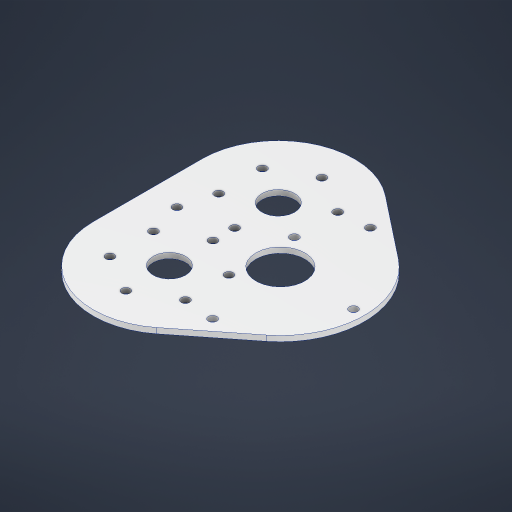
# Autodesk Inventor part: Gearboxes_3_thingy that holds motors and more
Saved by Autodesk Inventor 2024.4 (Build 284460000, 460)
## iProperties
Created: 2026-06-11
Part Number: Gearboxes_3_thingy that holds motors and more
Material: Aluminum 6061
Document SubType Name: Modeling
Designer: stanr
Density: 2.7 g/cm^3
Appearance: Aluminum - Flat
Author: stanr
Autodesk Inventor part; units mm, degrees
ref_plane "YZ Plane" through (0, 0, 0) normal (1, 0, 0) x (0, 1, 0)
ref_plane "XZ Plane" through (0, 0, 0) normal (0, 1, 0) x (-1, 0, 0)
ref_plane "XY Plane" through (0, 0, 0) normal (0, 0, 1) x (1, 0, 0)
sketch "Sketch1" plane through (0, 0, 0) normal (0, 1, 0) x (-1, 0, 0)
  circle A0 centre (0, 0) radius 31.75 construction
  circle A1 centre (0, -63.5) radius 31.75 construction
  circle A2 centre (0, 0) radius 9.525
  circle A3 centre (0, -63.5) radius 9.525
  circle A4 centre (0, 0) radius 25.4 construction
  circle A5 centre (0, -63.5) radius 25.4 construction
  circle A6 centre (0, 25.4) radius 2.4892
  circle A7 centre (-21.997, 12.7) radius 2.4892
  circle A8 centre (-21.997, -12.7) radius 2.4892
  circle A9 centre (0, -25.4) radius 2.4892
  circle A10 centre (21.997, -12.7) radius 2.4892
  circle A11 centre (21.997, 12.7) radius 2.4892
  circle A12 centre (0, -88.9) radius 2.4892
  circle A13 centre (21.997, -76.2) radius 2.4892
  circle A14 centre (21.997, -50.8) radius 2.4892
  circle A15 centre (0, -38.1) radius 2.4892
  circle A16 centre (-21.997, -50.8) radius 2.4892
  circle A17 centre (-21.997, -76.2) radius 2.4892
  circle A18 centre (-32.9859, -31.75) radius 36.2585 construction
  circle A19 centre (-32.9859, -31.75) radius 14.2875
  circle A20 centre (0, -63.5) radius 44.45
  circle A21 centre (0, 0) radius 44.45
  circle A22 centre (-32.9859, -31.75) radius 48.9585
  circle A23 centre (-39.4239, 14.2199) radius 2.4892
  circle A24 centre (-39.4239, 14.2199) radius 6.35 construction
  line L0 (-29.8666, 10.7726) -> (-33.4506, 12.0653) construction
  line L1 (-38.5432, 7.9312) -> (-38.0147, 4.1581) construction
  circle A25 centre (-39.4239, -77.7199) radius 2.4892
  circle A26 centre (-39.4239, -77.7199) radius 6.35 construction
  line L2 (-33.4506, -75.5653) -> (-29.8666, -74.2726) construction
  line L3 (-38.5432, -71.4312) -> (-38.0147, -67.6581) construction
  circle A27 centre (27.3566, -31.75) radius 2.4892
  circle A28 centre (27.3566, -31.75) radius 6.35 construction
  line L4 (23.2117, -26.9394) -> (20.7247, -24.053) construction
  line L5 (23.2117, -36.5606) -> (20.7247, -39.447) construction
  line L6 (44.45, 0) -> (44.45, -63.5)
  line L7 (-27.5218, 34.9049) -> (-63.2991, 6.6953)
  line L8 (-63.2991, -70.1953) -> (-27.5218, -98.4049)
  circle A29 centre (-75.5944, -31.75) radius 6.35 construction
  circle A30 centre (-75.5944, -31.75) radius 2.4892
  point P0 (31.1085, -31.75)
  dimension "d4" = 50.8
  dimension "d0" = 63.5
  dimension "d2" = 19.05
  dimension "d5" = 4.9784
  dimension "d8" = 360
  dimension "d12" = 360
  dimension "d14" = 72.517
  dimension "d15" = 28.575
  dimension "d38" = 45.7835
  dimension "d39" = 12.7
  dimension "d40" = 12.7
  dimension "d41" = 12.7
  dimension "d42" = 4.9784
  dimension "d43" = 12.7
  dimension "d44" = 3.81
  constraints: 29 centre point, 18 end point, 18 point on circle, 12 point on line, 10 coincident, 10 tangent, 9 equal radius, 5 equal length, 5 vertical alignment, 1 horizontal alignment, 30 other
  measures "d0" diameter of A0
  measures "d2" diameter of A2
  measures "d5" diameter of A6
  measures "d14" diameter of A18
  measures "d15" diameter of A19
  measures "d38" distance of point (0, 0) A18.centre
  measures "d39" radial gap between concentric circles of A1 A20
  measures "d40" radial gap between concentric circles of A0 A21
  measures "d41" radial gap between concentric circles of A18 A22
  measures "d42" diameter of A23
  measures "d43" diameter of A24
  measures "d44" distance of L0.start L0.end
extrude "Extrusion2" add sketch "Sketch1" along normal blind 3.175 contours A2 A22 A21 A20 | A2 A22 A20 A19 A21 | A22 L7 A21 | A21 A19 A20 A22 | A22 A21 A19 A20 | A20 A21 A22 | A21 L6 A20 | A20 A22 A3 A21 | A19 A21 A22 A3 A20 | A22 A20 L8
body "Solid2"
